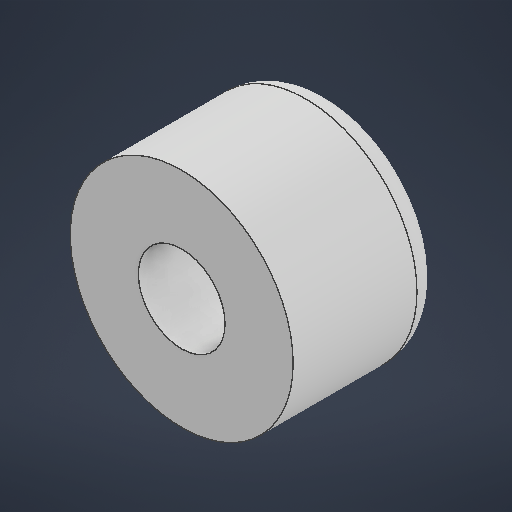
# Autodesk Inventor part: Стопор
Saved by Autodesk Inventor 2025 (Build 290162010, 162A)
## iProperties
Created: 2025-01-30
Part Number: Стопор
Material: Типовые
Document SubType Name: Modeling
Designer: Edward_Higgins
Density: 1 g/cm^3
Appearance: По умолчанию
Author: Edward_Higgins
Autodesk Inventor part; units mm, degrees
ref_plane "YZ Plane" through (0, 0, 0) normal (1, 0, 0) x (0, 1, 0)
ref_plane "XZ Plane" through (0, 0, 0) normal (0, 1, 0) x (-1, 0, 0)
ref_plane "XY Plane" through (0, 0, 0) normal (0, 0, 1) x (1, 0, 0)
sketch "Эскиз1" plane through (0, 0, 0) normal (0, 0, 1) x (1, 0, 0)
  circle A0 centre (0, 0) radius 4.5
  circle A1 centre (0, 0) radius 1.75
  line L0 (0, 3.4641) -> (3, 1.7321)
  line L1 (3, 1.7321) -> (3, -1.7321)
  line L2 (3, -1.7321) -> (0, -3.4641)
  line L3 (0, -3.4641) -> (-3, -1.7321)
  line L4 (-3, -1.7321) -> (-3, 1.7321)
  line L5 (-3, 1.7321) -> (0, 3.4641)
  dimension "d0" = 3.5
  dimension "d1" = 9
  dimension "d3" = 6
  constraints: 12 end point, 3 coincident, 2 centre point, 1 vertical, 13 other
  measures "d0" diameter of A1
  measures "d1" diameter of A0
  measures "d3" distance between parallel lines of L4 L1
extrude "Выдавливание1" add sketch "Эскиз1" along normal blind 6 contours A0 | L0 L1 L2 L3 L4 L5
extrude "Выдавливание2" cut sketch "Эскиз1" along normal blind 3.5 contours L0 L1 L2 L3 L4 L5
fillet "Сопряжение1" radius 1 1 edges at (-4.5, 0, 0)
